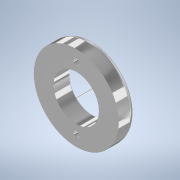
# Autodesk Inventor part: wheel_washer
Saved by Autodesk Inventor 2020 (Build 240168000, 168)
## iProperties
Created: 2015-12-06
Part Number: wheel_washer
Material: Aluminio 6061
Document SubType Name: Modeling
Designer: MIGUEL ANGEL
Density: 2.7 g/cm^3
Appearance: Cromo - Pulido
Author: MIGUEL ANGEL
Autodesk Inventor part; units mm, degrees
ref_plane "YZ Plane" through (0, 0, 0) normal (1, 0, 0) x (0, 1, 0)
ref_plane "XZ Plane" through (0, 0, 0) normal (0, 1, 0) x (-1, 0, 0)
ref_plane "XY Plane" through (0, 0, 0) normal (0, 0, 1) x (1, 0, 0)
sketch "Boceto1" plane through (0, 0, 0) normal (0, 1, 0) x (-1, 0, 0)
  circle A0 centre (0, 0) radius 15
  dimension "d0" = 30
  constraints: 1 centre point
  measures "d0" diameter of A0
extrude "Extrusión1" add sketch "Boceto1" along normal blind 6
sketch "Boceto2" plane through (0, 0, 0) normal (0, -1, 0) x (1, 0, 0)
  circle A0 centre (0, 0) radius 8
  dimension "d3" = 16
  constraints: 1 centre point, 1 coincident
  measures "d3" diameter of A0
extrude "Extrusión2" cut sketch "Boceto2" against normal through all
fillet "Empalme1" radius 2 1 edges at (15, 6, 0)
chamfer "Chaflán1" distance 0.5 angle 45 1 edges at (-8, 6, 0)
sketch "Boceto3" plane through (0, 6, 0) normal (0, 1, 0) x (1, 0, 0)
  circle A0 centre (0, 0) radius 13 projected
  circle A1 centre (0, 0) radius 11 construction
  point P0 (0, 11)
  point P1 (0, -11)
  dimension "d10" = 2
  constraints: 2 point on circle, 1 centre point
  measures "d10" radial gap between concentric circles of A0 A1
hole "Agujero1" at (0, 6, -11) at (0, 6, 11) direction (0, -1, 0) diameter 2 end through all
